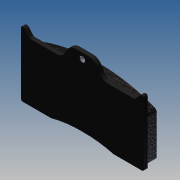
# Autodesk Inventor part: BRAKE PAD
Saved by Autodesk Inventor 2012 SP1 (Build 160190100, 190)
## iProperties
Created: 2012-02-16
Part Number: BRAKE PAD
Project: Alpha
Material: Acier
Document SubType Name: Modeling
Designer: A.COMEAU
Density: 7.85 g/cm^3
Author: A.COMEAU
Autodesk Inventor part; units mm, degrees
ref_plane "YZ Plane" through (0, 0, 0) normal (1, 0, 0) x (0, 1, 0)
ref_plane "XZ Plane" through (0, 0, 0) normal (0, 1, 0) x (-1, 0, 0)
ref_plane "XY Plane" through (0, 0, 0) normal (0, 0, 1) x (1, 0, 0)
sketch "Esquisse1" plane through (0, 0, 0) normal (0, 0, 1) x (1, 0, 0)
  line L0 (-186.69, 0) -> (186.69, 0) projected
  line L1 (0, -197.485) -> (0, 251.46) projected
  circle A0 centre (0, 0) radius 133.35 construction
  line L2 (-50.292, 138.9194) -> (-50.292, 88.9302)
  line L3 (50.292, 88.9302) -> (50.292, 138.9194)
  line L4 (-5.4717, 146.4909) -> (0, 146.4909)
  line L5 (-59.3639, 174.3189) -> (62.2899, 174.3189) construction
  line L6 (62.2899, 174.3189) -> (62.2899, 74.4875) construction
  line L7 (62.2899, 74.4875) -> (-59.3639, 74.4875) construction
  line L8 (-59.3639, 74.4875) -> (-59.3639, 174.3189) construction
  line L9 (-46.6745, 139.3954) -> (-43.813, 136.0491)
  line L10 (-41.4, 134.9375) -> (-21.2184, 134.9375)
  line L11 (-14.2687, 139.0403) -> (-12.4215, 142.3881)
  line L12 (0, 14.2875) -> (0, 187.325) construction
  arc A1 (-46.6745, 139.3954) -> (-48.8631, 140.499) centre (-49.0875, 137.3319) ccw
  arc A2 (-43.813, 136.0491) -> (-41.4, 134.9375) centre (-41.4, 138.1125) ccw
  arc A3 (-48.8631, 140.499) -> (-50.292, 138.9194) centre (-48.7045, 138.9194) ccw
  arc A4 (-21.2184, 134.9375) -> (-14.2687, 139.0403) centre (-21.2184, 142.875) ccw
  arc A5 (-5.4717, 146.4909) -> (-12.4215, 142.3881) centre (-5.4717, 138.5534) ccw
  line L13 (5.4717, 146.4909) -> (0, 146.4909)
  line L14 (46.6745, 139.3954) -> (43.813, 136.0491)
  line L15 (41.4, 134.9375) -> (21.2184, 134.9375)
  line L16 (14.2687, 139.0403) -> (12.4215, 142.3881)
  arc A6 (48.8631, 140.499) -> (46.6745, 139.3954) centre (49.0875, 137.3319) ccw
  arc A7 (41.4, 134.9375) -> (43.813, 136.0491) centre (41.4, 138.1125) ccw
  arc A8 (50.292, 138.9194) -> (48.8631, 140.499) centre (48.7045, 138.9194) ccw
  arc A9 (14.2687, 139.0403) -> (21.2184, 134.9375) centre (21.2184, 142.875) ccw
  arc A10 (12.4215, 142.3881) -> (5.4717, 146.4909) centre (5.4717, 138.5534) ccw
  line L17 (-48.7045, 87.3427) -> (-25.6128, 87.3427)
  arc A11 (0, 90.4875) -> (-25.1966, 87.3982) centre (-1.8902, 1.6076) ccw
  arc A12 (-50.292, 88.9302) -> (-48.7045, 87.3427) centre (-48.7045, 88.9302) ccw
  arc A13 (-25.6128, 87.3427) -> (-25.1966, 87.3982) centre (-25.6128, 88.9302) ccw
  line L18 (48.7045, 87.3427) -> (25.6128, 87.3427)
  arc A14 (25.1966, 87.3982) -> (0, 90.4875) centre (1.8902, 1.6076) ccw
  arc A15 (25.1966, 87.3982) -> (25.6128, 87.3427) centre (25.6128, 88.9302) ccw
  arc A16 (48.7045, 87.3427) -> (50.292, 88.9302) centre (48.7045, 88.9302) ccw
  point P0 (-25.4, 87.3427)
  point P1 (48.7045, 87.3427)
  dimension "d0" = 266.7
  dimension "d1" = 100.584
  dimension "d37" = 121.6538
  dimension "d38" = 99.8314
  dimension "d39" = 74.4875
  dimension "d40" = 59.3639
  dimension "d52" = 3.175
  dimension "d55" = 1.5875
  dimension "d58" = 7.9375
  dimension "d67" = 88.9
  dimension "d68" = 1.5875
  dimension "d72" = 1.5875
  constraints: 33 point on circle, 26 end point, 19 symmetric about line, 17 centre point, 14 tangent, 6 point on line, 3 equal radius, 3 parallel, 1 coincident, 10 other
  measures "d0" diameter of A0
  measures "d1" distance between parallel lines of L3 L2
  measures "d37" distance of L5.start L5.end
  measures "d38" distance of L5.end L6.end
  measures "d39" distance between parallel lines of L0 L7
  measures "d40" distance between parallel lines of L1 L8
  measures "d52" radius of A1
  measures "d55" radius of A3
  measures "d58" radius of A4
  measures "d67" radius of A11
  measures "d68" radius of A12
  measures "d72" radius of A16
extrude "Extrusion1" add sketch "Esquisse1" along normal blind 3.175
sketch "Esquisse2" plane through (0, 0, 0) normal (0, 0, -1) x (-1, 0, 0)
  line L0 (-50.292, 138.9194) -> (-50.292, 88.9302) projected
  line L1 (-21.2184, 134.9375) -> (-41.4, 134.9375) projected
  line L2 (-48.2586, 90.2748) -> (-48.2586, 122.0318)
  line L3 (-46.6734, 88.6873) -> (-26.9271, 88.6585)
  arc A0 (0, 91.9607) -> (-26.9271, 88.6585) centre (1.948, -35.3617) ccw
  arc A1 (0, 133.35) -> (-46.2034, 125.0028) centre (-0.3874, 3.4484) ccw
  line L4 (0, -197.485) -> (0, 251.46) projected
  line L5 (48.2586, 90.2748) -> (48.2586, 122.0318)
  line L6 (46.6734, 88.6873) -> (27.1101, 88.6588)
  arc A2 (26.75, 88.6996) -> (0, 91.9607) centre (-1.948, -35.3617) ccw
  arc A3 (46.2034, 125.0028) -> (0, 133.35) centre (0.3874, 3.4484) ccw
  arc A4 (-48.2586, 90.2748) -> (-46.6734, 88.6873) centre (-46.6711, 90.2748) ccw
  arc A5 (26.75, 88.6996) -> (27.1101, 88.6588) centre (27.1078, 90.2463) ccw
  arc A6 (46.6734, 88.6873) -> (48.2586, 90.2748) centre (46.6711, 90.2748) ccw
  arc A7 (-46.2034, 125.0028) -> (-48.2586, 122.0318) centre (-45.0836, 122.0318) ccw
  arc A8 (48.2586, 122.0318) -> (46.2034, 125.0028) centre (45.0836, 122.0318) ccw
  point P0 (0, 0)
  point P1 (-48.2586, 88.6897)
  point P2 (-48.2586, 124.2082)
  point P3 (48.2586, 88.6897)
  point P4 (48.2586, 124.2082)
  point P5 (26.9271, 88.6585)
  dimension "d80" = 1.5875
  dimension "d81" = 3.175
  constraints: 21 point on circle, 10 tangent, 9 centre point, 8 end point, 7 point on line, 5 symmetric about line, 3 equal radius, 1 parallel, 1 perpendicular, 2 other
  measures "d80" radius of A4
  measures "d81" radius of A7
extrude "Extrusion2" add sketch "Esquisse2" along normal blind 9.271
sketch "Esquisse3" plane through (0, 0, 0) normal (0, 0, -1) x (-1, 0, 0)
  circle A0 centre (0, 141.7847) radius 2.1822
  point P0 (0, 0)
  constraints: 1 centre point
extrude "Extrusion3" cut sketch "Esquisse3" against normal blind 9.271
equation "\"d0\" = para_d"
equation "\"para_a\" = 25.4"
equation "\"para_b\" = 25.4"
equation "\"para_c\" = 25.4"
equation "\"para_d\" = 266.7"
equation "\"para_e\" = 25.4"
